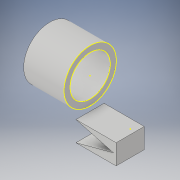
# Autodesk Inventor part: Whistle Cutout
Saved by Autodesk Inventor 2019 (Build 230136000, 136)
## iProperties
Created: 2019-01-22
Part Number: Whistle Cutout
Material: Generic
Document SubType Name: Modeling
Designer: Kepler
Density: 1 g/cm^3
Appearance: Default
Author: Kepler
Autodesk Inventor part; units mm, degrees
ref_plane "YZ Plane" through (0, 0, 0) normal (1, 0, 0) x (0, 1, 0)
ref_plane "XZ Plane" through (0, 0, 0) normal (0, 1, 0) x (-1, 0, 0)
ref_plane "XY Plane" through (0, 0, 0) normal (0, 0, 1) x (1, 0, 0)
sketch "Sketch1" plane through (0, 0, 0) normal (0, 0, 1) x (1, 0, 0)
  line L0 (0, 0) -> (20, 0)
  line L1 (0, 0) -> (0, 3)
  line L2 (0, 3) -> (20, 3)
  line L3 (20, 3) -> (20, 0)
  line L4 (20, 13) -> (0, 13)
  dimension "d1" = 3
  dimension "d2" = 20
  dimension "d3" = 10
  dimension "d4" = 20
  dimension "d5" = 20
  constraints: 10 end point, 2 perpendicular, 1 horizontal, 1 parallel, 1 vertical
  measures "d1" distance of L0.start L1.end
  measures "d2" distance of L1.end L2.end
  measures "d3" distance of L2.end L4.start
  measures "d4" distance of L4.start L4.end
  measures "d5" diameter of L2 L4
revolve "Revolution1" add sketch "Sketch1" angle 360 about axis through (20, 13, 0) along (-1, 0, 0)
sketch "Sketch3" plane through (0, 13, 0) normal (-1, 0, 0) x (0, 0, 1)
  point P0 (0, -13)
sketch "Sketch4" plane through (20, 13, 0) normal (1, 0, 0) x (0, 0, -1)
  circle A0 centre (0, 0) radius 10 projected
  circle A1 centre (0, 0) radius 13 projected
sketch "Sketch5" plane through (20, 13, 0) normal (1, 0, 0) x (0, 0, -1)
  point P0 (0, -13)
sketch "Sketch6" plane through (20, 13, 0) normal (1, 0, 0) x (0, 0, -1)
  circle A0 centre (0, 0) radius 13 projected
  circle A1 centre (0, 0) radius 10 projected
  line L0 (-7, -15.4207) -> (-7, -25.4207)
  line L1 (-7, -25.4207) -> (7, -25.4207)
  line L2 (7, -25.4207) -> (7, -15.4207)
  line L3 (-7, -15.4207) -> (7, -15.4207)
  point P0 (0, -13)
  dimension "d20" = 10
  dimension "d21" = 14
  constraints: 8 end point, 2 perpendicular, 1 horizontal, 1 vertical alignment
  measures "d20" distance of L0.start L0.end
  measures "d21" distance of L0.end L1.end
extrude "Extrusion1" add sketch "Sketch6" along normal blind 20 contours L3 L2 L1 L0
sketch "Sketch7" plane through (20, -12.4207, -7) normal (0, 0, -1) x (-1, 0, 0)
  line L0 (0, 10) -> (0, 0) projected
  line L1 (0, 0) -> (-18.6603, 5)
  line L2 (0, 10) -> (-20, 10) projected
  line L3 (-18.6603, 5) -> (0, 10)
  line L4 (0, 0) -> (-20, 0) projected
  point P0 (20, 12.4207)
  dimension "d24" = 15
  dimension "d25" = 15
  constraints: 4 end point
  measures "d24" angle of L4 L1
  measures "d25" angle of L2 L3
extrude "Extrusion2" cut sketch "Sketch7" against normal blind 14
sketch "Sketch8" plane through (40, 13, 0) normal (1, 0, 0) x (0, 0, -1)
  point P0 (0, -13)
sketch "Sketch9" plane through (20, 13, 0) normal (1, 0, 0) x (0, 0, -1)
  point P0 (0, -13)
equation "\"d25\" = d24"
body "Solid1"
